Autodesk Inventor part; units mm, degrees
(part 3 of 4)
  spline S198 degree 3 poles (-4.8758, 47.2578) (-4.8804, 47.27) (-4.8822, 47.8237) (-4.8797, 48.4882) knots 0 0 0 0 1 1 1 1
  line L1039 (-4.8758, 47.2578) -> (-4.8804, 47.27) construction
  line L1040 (-4.8804, 47.27) -> (-4.8822, 47.8237) construction
  line L1041 (-4.8822, 47.8237) -> (-4.8797, 48.4882) construction
  line L1042 (-4.8797, 48.4882) -> (-4.8751, 49.6965)
  line L1043 (-4.8751, 49.6965) -> (-4.8001, 49.7019)
  line L1044 (-4.8001, 49.7019) -> (-4.7252, 49.7073)
  line L1045 (-4.7252, 49.7073) -> (-4.7252, 48.5423)
  line L1046 (-4.7252, 48.5423) -> (-4.7252, 47.3772)
  line L1047 (-4.7252, 47.3772) -> (-3.5301, 47.3727)
  line L1048 (-3.5301, 47.3727) -> (-2.3351, 47.3681)
  line L1049 (-2.3351, 47.3681) -> (-2.3351, 47.3064)
  line L1050 (-2.3351, 47.3064) -> (-2.3351, 47.2447)
  line L1051 (-2.3351, 47.2447) -> (-3.6012, 47.2402)
  spline S199 degree 3 poles (-3.6012, 47.2402) (-4.6047, 47.2365) (-4.8691, 47.2402) (-4.8758, 47.2578) knots 11 11 11 11 12 12 12 12
  line L1052 (-3.6012, 47.2402) -> (-4.6047, 47.2365) construction
  line L1053 (-4.6047, 47.2365) -> (-4.8691, 47.2402) construction
  line L1054 (-4.8691, 47.2402) -> (-4.8758, 47.2578) construction
  spline S200 degree 3 poles (-2.2078, 47.2468) (-2.2287, 47.2677) (-2.2232, 49.7053) (-2.2023, 49.7053) (-2.1923, 49.7053) (-2.134, 49.6636) (-2.0728, 49.6127) knots 0 0 0 0 1 1 1 2 2 2 2
  line L1055 (-2.2078, 47.2468) -> (-2.2287, 47.2677) construction
  line L1056 (-2.2287, 47.2677) -> (-2.2232, 49.7053) construction
  line L1057 (-2.2232, 49.7053) -> (-2.2023, 49.7053) construction
  line L1058 (-2.2023, 49.7053) -> (-2.1923, 49.7053) construction
  line L1059 (-2.1923, 49.7053) -> (-2.134, 49.6636) construction
  line L1060 (-2.134, 49.6636) -> (-2.0728, 49.6127) construction
  spline S201 degree 3 poles (-2.0728, 49.6127) (-2.0116, 49.5618) (-1.7837, 49.3794) (-1.5662, 49.2075) knots 2 2 2 2 3 3 3 3
  line L1061 (-2.0728, 49.6127) -> (-2.0116, 49.5618) construction
  line L1062 (-2.0116, 49.5618) -> (-1.7837, 49.3794) construction
  line L1063 (-1.7837, 49.3794) -> (-1.5662, 49.2075) construction
  spline S202 degree 3 poles (-1.5662, 49.2075) (-1.3488, 49.0356) (-1.1154, 48.851) (-1.0475, 48.7972) knots 3 3 3 3 4 4 4 4
  line L1064 (-1.5662, 49.2075) -> (-1.3488, 49.0356) construction
  line L1065 (-1.3488, 49.0356) -> (-1.1154, 48.851) construction
  line L1066 (-1.1154, 48.851) -> (-1.0475, 48.7972) construction
  spline S203 degree 3 poles (-1.0475, 48.7972) (-0.9795, 48.7435) (-0.9144, 48.7016) (-0.9026, 48.7041) knots 4 4 4 4 5 5 5 5
  line L1067 (-1.0475, 48.7972) -> (-0.9795, 48.7435) construction
  line L1068 (-0.9795, 48.7435) -> (-0.9144, 48.7016) construction
  line L1069 (-0.9144, 48.7016) -> (-0.9026, 48.7041) construction
  spline S204 degree 3 poles (-0.9026, 48.7041) (-0.8827, 48.7084) (-0.2139, 49.2329) (0.0269, 49.4331) knots 5 5 5 5 6 6 6 6
  line L1070 (-0.9026, 48.7041) -> (-0.8827, 48.7084) construction
  line L1071 (-0.8827, 48.7084) -> (-0.2139, 49.2329) construction
  line L1072 (-0.2139, 49.2329) -> (0.0269, 49.4331) construction
  spline S205 degree 3 poles (0.0269, 49.4331) (0.2602, 49.6271) (0.373, 49.7068) (0.3818, 49.6839) knots 6 6 6 6 7 7 7 7
  line L1073 (0.0269, 49.4331) -> (0.2602, 49.6271) construction
  line L1074 (0.2602, 49.6271) -> (0.373, 49.7068) construction
  line L1075 (0.373, 49.7068) -> (0.3818, 49.6839) construction
  spline S206 degree 3 poles (0.3818, 49.6839) (0.3865, 49.6714) (0.3884, 49.1175) (0.3859, 48.4529) knots 7 7 7 7 8 8 8 8
  line L1076 (0.3818, 49.6839) -> (0.3865, 49.6714) construction
  line L1077 (0.3865, 49.6714) -> (0.3884, 49.1175) construction
  line L1078 (0.3884, 49.1175) -> (0.3859, 48.4529) construction
  line L1079 (0.3859, 48.4529) -> (0.3813, 47.2447)
  line L1080 (0.3813, 47.2447) -> (0.3196, 47.2447)
  line L1081 (0.3196, 47.2447) -> (0.2578, 47.2447)
  line L1082 (0.2578, 47.2447) -> (0.249, 48.3248)
  line L1083 (0.249, 48.3248) -> (0.2402, 49.4049)
  line L1084 (0.2402, 49.4049) -> (0.0991, 49.2937)
  spline S207 degree 3 poles (0.0991, 49.2937) (-0.7488, 48.6253) (-0.8829, 48.5235) (-0.9156, 48.5235) (-0.9275, 48.5235) (-1.0142, 48.585) (-1.1083, 48.6602) knots 14 14 14 14 15 15 15 16 16 16 16
  line L1085 (0.0991, 49.2937) -> (-0.7488, 48.6253) construction
  line L1086 (-0.7488, 48.6253) -> (-0.8829, 48.5235) construction
  line L1087 (-0.8829, 48.5235) -> (-0.9156, 48.5235) construction
  line L1088 (-0.9156, 48.5235) -> (-0.9275, 48.5235) construction
  line L1089 (-0.9275, 48.5235) -> (-1.0142, 48.585) construction
  line L1090 (-1.0142, 48.585) -> (-1.1083, 48.6602) construction
  spline S208 degree 3 poles (-1.1083, 48.6602) (-1.2024, 48.7354) (-1.3813, 48.8763) (-1.5057, 48.9733) knots 16 16 16 16 17 17 17 17
  line L1091 (-1.1083, 48.6602) -> (-1.2024, 48.7354) construction
  line L1092 (-1.2024, 48.7354) -> (-1.3813, 48.8763) construction
  line L1093 (-1.3813, 48.8763) -> (-1.5057, 48.9733) construction
  spline S209 degree 3 poles (-1.5057, 48.9733) (-1.6302, 49.0703) (-1.8082, 49.2104) (-1.9013, 49.2847) knots 17 17 17 17 18 18 18 18
  line L1094 (-1.5057, 48.9733) -> (-1.6302, 49.0703) construction
  line L1095 (-1.6302, 49.0703) -> (-1.8082, 49.2104) construction
  line L1096 (-1.8082, 49.2104) -> (-1.9013, 49.2847) construction
  line L1097 (-1.9013, 49.2847) -> (-2.0705, 49.4197)
  line L1098 (-2.0705, 49.4197) -> (-2.0793, 48.3322)
  line L1099 (-2.0793, 48.3322) -> (-2.0882, 47.2447)
  line L1100 (-2.0882, 47.2447) -> (-2.1417, 47.2394)
  spline S210 degree 3 poles (-2.1417, 47.2394) (-2.1712, 47.2365) (-2.2009, 47.2398) (-2.2078, 47.2468) knots 22 22 22 22 23 23 23 23
  line L1101 (-2.1417, 47.2394) -> (-2.1712, 47.2365) construction
  line L1102 (-2.1712, 47.2365) -> (-2.2009, 47.2398) construction
  line L1103 (-2.2009, 47.2398) -> (-2.2078, 47.2468) construction
  spline S211 degree 3 poles (0.504, 47.2579) (0.4994, 47.27) (0.4977, 47.8237) (0.5002, 48.4882) knots 0 0 0 0 1 1 1 1
  line L1104 (0.504, 47.2579) -> (0.4994, 47.27) construction
  line L1105 (0.4994, 47.27) -> (0.4977, 47.8237) construction
  line L1106 (0.4977, 47.8237) -> (0.5002, 48.4882) construction
  line L1107 (0.5002, 48.4882) -> (0.5048, 49.6965)
  line L1108 (0.5048, 49.6965) -> (1.7615, 49.701)
  line L1109 (1.7615, 49.701) -> (3.0183, 49.7055)
  line L1110 (3.0183, 49.7055) -> (3.0183, 49.6437)
  spline S212 degree 3 poles (3.0183, 49.6437) (3.0183, 49.6061) (3.0096, 49.5817) (2.9962, 49.5816) knots 5 5 5 5 6 6 6 6
  line L1111 (3.0183, 49.6437) -> (3.0183, 49.6061) construction
  line L1112 (3.0183, 49.6061) -> (3.0096, 49.5817) construction
  line L1113 (3.0096, 49.5817) -> (2.9962, 49.5816) construction
  spline S213 degree 3 poles (2.9962, 49.5816) (2.9841, 49.5814) (2.4444, 49.5816) (1.7968, 49.5818) knots 6 6 6 6 7 7 7 7
  line L1114 (2.9962, 49.5816) -> (2.9841, 49.5814) construction
  line L1115 (2.9841, 49.5814) -> (2.4444, 49.5816) construction
  line L1116 (2.4444, 49.5816) -> (1.7968, 49.5818) construction
  line L1117 (1.7968, 49.5818) -> (0.6194, 49.5823)
  line L1118 (0.6194, 49.5823) -> (0.6194, 49.0617)
  line L1119 (0.6194, 49.0617) -> (0.6194, 48.5411)
  line L1120 (0.6194, 48.5411) -> (1.8188, 48.5411)
  line L1121 (1.8188, 48.5411) -> (3.0183, 48.5411)
  line L1122 (3.0183, 48.5411) -> (3.0183, 48.4813)
  spline S214 degree 3 poles (3.0183, 48.4813) (3.0183, 48.443) (3.0083, 48.4176) (2.9904, 48.4107) knots 13 13 13 13 14 14 14 14
  line L1123 (3.0183, 48.4813) -> (3.0183, 48.443) construction
  line L1124 (3.0183, 48.443) -> (3.0083, 48.4176) construction
  line L1125 (3.0083, 48.4176) -> (2.9904, 48.4107) construction
  spline S215 degree 3 poles (2.9904, 48.4107) (2.9751, 48.4048) (2.4353, 48.4) (1.791, 48.4) knots 14 14 14 14 15 15 15 15
  line L1126 (2.9904, 48.4107) -> (2.9751, 48.4048) construction
  line L1127 (2.9751, 48.4048) -> (2.4353, 48.4) construction
  line L1128 (2.4353, 48.4) -> (1.791, 48.4) construction
  line L1129 (1.791, 48.4) -> (0.6194, 48.4)
  line L1130 (0.6194, 48.4) -> (0.6194, 47.8885)
  line L1131 (0.6194, 47.8885) -> (0.6194, 47.377)
  line L1132 (0.6194, 47.377) -> (1.791, 47.377)
  spline S216 degree 3 poles (1.791, 47.377) (2.4353, 47.377) (2.9751, 47.3721) (2.9904, 47.3663) knots 19 19 19 19 20 20 20 20
  line L1133 (1.791, 47.377) -> (2.4353, 47.377) construction
  line L1134 (2.4353, 47.377) -> (2.9751, 47.3721) construction
  line L1135 (2.9751, 47.3721) -> (2.9904, 47.3663) construction
  spline S217 degree 3 poles (2.9904, 47.3663) (3.0066, 47.36) (3.0183, 47.3349) (3.0183, 47.3064) (3.0183, 47.2779) (3.0066, 47.2528) (2.9904, 47.2466) knots 20 20 20 20 21 21 21 22 22 22 22
  line L1136 (2.9904, 47.3663) -> (3.0066, 47.36) construction
  line L1137 (3.0066, 47.36) -> (3.0183, 47.3349) construction
  line L1138 (3.0183, 47.3349) -> (3.0183, 47.3064) construction
  line L1139 (3.0183, 47.3064) -> (3.0183, 47.2779) construction
  line L1140 (3.0183, 47.2779) -> (3.0066, 47.2528) construction
  line L1141 (3.0066, 47.2528) -> (2.9904, 47.2466) construction
  spline S218 degree 3 poles (2.9904, 47.2466) (2.9751, 47.2407) (2.4112, 47.2359) (1.7375, 47.2359) (0.7737, 47.2359) (0.5107, 47.2405) (0.504, 47.2579) knots 22 22 22 22 23 23 23 24 24 24 24
  line L1142 (2.9904, 47.2466) -> (2.9751, 47.2407) construction
  line L1143 (2.9751, 47.2407) -> (2.4112, 47.2359) construction
  line L1144 (2.4112, 47.2359) -> (1.7375, 47.2359) construction
  line L1145 (1.7375, 47.2359) -> (0.7737, 47.2359) construction
  line L1146 (0.7737, 47.2359) -> (0.5107, 47.2405) construction
  line L1147 (0.5107, 47.2405) -> (0.504, 47.2579) construction
  line L1148 (0.504, 47.2579) -> (0.504, 47.2579)
  spline S219 degree 3 poles (5.3893, 47.496) (5.2553, 47.6391) (5.0332, 47.8753) (4.8957, 48.0208) knots 0 0 0 0 1 1 1 1
  line L1149 (5.3893, 47.496) -> (5.2553, 47.6391) construction
  line L1150 (5.2553, 47.6391) -> (5.0332, 47.8753) construction
  line L1151 (5.0332, 47.8753) -> (4.8957, 48.0208) construction
  spline S220 degree 3 poles (4.8957, 48.0208) (4.7582, 48.1663) (4.6241, 48.3111) (4.5979, 48.3425) knots 1 1 1 1 2 2 2 2
  line L1152 (4.8957, 48.0208) -> (4.7582, 48.1663) construction
  line L1153 (4.7582, 48.1663) -> (4.6241, 48.3111) construction
  line L1154 (4.6241, 48.3111) -> (4.5979, 48.3425) construction
  line L1155 (4.5979, 48.3425) -> (4.5501, 48.3996)
  line L1156 (4.5501, 48.3996) -> (3.8592, 48.4042)
  line L1157 (3.8592, 48.4042) -> (3.1682, 48.4088)
  line L1158 (3.1682, 48.4088) -> (3.1627, 48.475)
  line L1159 (3.1627, 48.475) -> (3.1573, 48.5411)
  line L1160 (3.1573, 48.5411) -> (4.4195, 48.5411)
  line L1161 (4.4195, 48.5411) -> (5.6818, 48.5411)
  line L1162 (5.6818, 48.5411) -> (5.6818, 49.0619)
  line L1163 (5.6818, 49.0619) -> (5.6818, 49.5827)
  line L1164 (5.6818, 49.5827) -> (4.425, 49.5811)
  line L1165 (4.425, 49.5811) -> (3.1682, 49.5796)
  line L1166 (3.1682, 49.5796) -> (3.1627, 49.6424)
  line L1167 (3.1627, 49.6424) -> (3.1573, 49.7053)
  line L1168 (3.1573, 49.7053) -> (4.4813, 49.7053)
  line L1169 (4.4813, 49.7053) -> (5.8052, 49.7053)
  line L1170 (5.8052, 49.7053) -> (5.8052, 49.0634)
  spline S221 degree 3 poles (5.8052, 49.0634) (5.8052, 48.4943) (5.8021, 48.4202) (5.7774, 48.4107) knots 18 18 18 18 19 19 19 19
  line L1171 (5.8052, 49.0634) -> (5.8052, 48.4943) construction
  line L1172 (5.8052, 48.4943) -> (5.8021, 48.4202) construction
  line L1173 (5.8021, 48.4202) -> (5.7774, 48.4107) construction
  spline S222 degree 3 poles (5.7774, 48.4107) (5.762, 48.4048) (5.5191, 48.4) (5.2376, 48.4) knots 19 19 19 19 20 20 20 20
  line L1174 (5.7774, 48.4107) -> (5.762, 48.4048) construction
  line L1175 (5.762, 48.4048) -> (5.5191, 48.4) construction
  line L1176 (5.5191, 48.4) -> (5.2376, 48.4) construction
  line L1177 (5.2376, 48.4) -> (4.7258, 48.4)
  line L1178 (4.7258, 48.4) -> (4.9612, 48.1488)
  spline S223 degree 3 poles (4.9612, 48.1488) (5.0907, 48.0107) (5.3149, 47.7706) (5.4593, 47.6153) knots 22 22 22 22 23 23 23 23
  line L1179 (4.9612, 48.1488) -> (5.0907, 48.0107) construction
  line L1180 (5.0907, 48.0107) -> (5.3149, 47.7706) construction
  line L1181 (5.3149, 47.7706) -> (5.4593, 47.6153) construction
  spline S224 degree 3 poles (5.4593, 47.6153) (5.6037, 47.4599) (5.7402, 47.3157) (5.7627, 47.2947) knots 23 23 23 23 24 24 24 24
  line L1182 (5.4593, 47.6153) -> (5.6037, 47.4599) construction
  line L1183 (5.6037, 47.4599) -> (5.7402, 47.3157) construction
  line L1184 (5.7402, 47.3157) -> (5.7627, 47.2947) construction
  spline S225 degree 3 poles (5.7627, 47.2947) (5.8098, 47.2508) (5.7917, 47.2358) (5.6912, 47.2358) (5.6388, 47.2358) (5.6079, 47.2625) (5.3893, 47.496) knots 24 24 24 24 25 25 25 26 26 26 26
  line L1185 (5.7627, 47.2947) -> (5.8098, 47.2508) construction
  line L1186 (5.8098, 47.2508) -> (5.7917, 47.2358) construction
  line L1187 (5.7917, 47.2358) -> (5.6912, 47.2358) construction
  line L1188 (5.6912, 47.2358) -> (5.6388, 47.2358) construction
  line L1189 (5.6388, 47.2358) -> (5.6079, 47.2625) construction
  line L1190 (5.6079, 47.2625) -> (5.3893, 47.496) construction
  spline S226 degree 3 poles (5.9356, 47.2609) (5.9303, 47.2748) (5.9285, 47.3046) (5.9317, 47.3272) knots 0 0 0 0 1 1 1 1
  line L1191 (5.9356, 47.2609) -> (5.9303, 47.2748) construction
  line L1192 (5.9303, 47.2748) -> (5.9285, 47.3046) construction
  line L1193 (5.9285, 47.3046) -> (5.9317, 47.3272) construction
  line L1194 (5.9317, 47.3272) -> (5.9375, 47.3681)
  line L1195 (5.9375, 47.3681) -> (7.1149, 47.3727)
  line L1196 (7.1149, 47.3727) -> (8.2923, 47.3772)
  line L1197 (8.2923, 47.3772) -> (8.2923, 47.8885)
  line L1198 (8.2923, 47.8885) -> (8.2923, 48.3998)
  line L1199 (8.2923, 48.3998) -> (7.1149, 48.4043)
  line L1200 (7.1149, 48.4043) -> (5.9375, 48.4088)
  line L1201 (5.9375, 48.4088) -> (5.9375, 49.0526)
  line L1202 (5.9375, 49.0526) -> (5.9375, 49.6965)
  line L1203 (5.9375, 49.6965) -> (7.1811, 49.6965)
  line L1204 (7.1811, 49.6965) -> (8.4246, 49.6965)
  line L1205 (8.4246, 49.6965) -> (8.4305, 49.6547)
  spline S227 degree 3 poles (8.4305, 49.6547) (8.4338, 49.6318) (8.4294, 49.606) (8.4207, 49.5973) knots 13 13 13 13 14 14 14 14
  line L1206 (8.4305, 49.6547) -> (8.4338, 49.6318) construction
  line L1207 (8.4338, 49.6318) -> (8.4294, 49.606) construction
  line L1208 (8.4294, 49.606) -> (8.4207, 49.5973) construction
  spline S228 degree 3 poles (8.4207, 49.5973) (8.4118, 49.5884) (7.8969, 49.5816) (7.2374, 49.5816) knots 14 14 14 14 15 15 15 15
  line L1209 (8.4207, 49.5973) -> (8.4118, 49.5884) construction
  line L1210 (8.4118, 49.5884) -> (7.8969, 49.5816) construction
  line L1211 (7.8969, 49.5816) -> (7.2374, 49.5816) construction
  line L1212 (7.2374, 49.5816) -> (6.0698, 49.5815)
  line L1213 (6.0698, 49.5815) -> (6.0698, 49.0615)
  line L1214 (6.0698, 49.0615) -> (6.0698, 48.5414)
  line L1215 (6.0698, 48.5414) -> (7.2472, 48.5368)
  line L1216 (7.2472, 48.5368) -> (8.4246, 48.5323)
  line L1217 (8.4246, 48.5323) -> (8.4246, 47.8885)
  line L1218 (8.4246, 47.8885) -> (8.4246, 47.2447)
  line L1219 (8.4246, 47.2447) -> (7.185, 47.2402)
  spline S229 degree 3 poles (7.185, 47.2402) (6.1218, 47.2363) (5.944, 47.2392) (5.9356, 47.2609) knots 23 23 23 23 24 24 24 24
  line L1220 (7.185, 47.2402) -> (6.1218, 47.2363) construction
  line L1221 (6.1218, 47.2363) -> (5.944, 47.2392) construction
  line L1222 (5.944, 47.2392) -> (5.9356, 47.2609) construction
  spline S230 degree 3 poles (-7.3426, 48.3876) (-7.3645, 48.4036) (-7.3721, 48.4285) (-7.368, 48.4714) knots 0 0 0 0 1 1 1 1
  line L1223 (-7.3426, 48.3876) -> (-7.3645, 48.4036) construction
  line L1224 (-7.3645, 48.4036) -> (-7.3721, 48.4285) construction
  line L1225 (-7.3721, 48.4285) -> (-7.368, 48.4714) construction
  line L1226 (-7.368, 48.4714) -> (-7.3622, 48.5323)
  line L1227 (-7.3622, 48.5323) -> (-6.3127, 48.5323)
  line L1228 (-6.3127, 48.5323) -> (-5.2632, 48.5323)
  line L1229 (-5.2632, 48.5323) -> (-5.2574, 48.4714)
  spline S231 degree 3 poles (-5.2574, 48.4714) (-5.2533, 48.4285) (-5.2609, 48.4036) (-5.2828, 48.3876) knots 5 5 5 5 6 6 6 6
  line L1230 (-5.2574, 48.4714) -> (-5.2533, 48.4285) construction
  line L1231 (-5.2533, 48.4285) -> (-5.2609, 48.4036) construction
  line L1232 (-5.2609, 48.4036) -> (-5.2828, 48.3876) construction
  spline S232 degree 3 poles (-5.2828, 48.3876) (-5.3285, 48.3541) (-7.2968, 48.3541) (-7.3426, 48.3876) knots 6 6 6 6 7 7 7 7
  line L1233 (-5.2828, 48.3876) -> (-5.3285, 48.3541) construction
  line L1234 (-5.3285, 48.3541) -> (-7.2968, 48.3541) construction
  line L1235 (-7.2968, 48.3541) -> (-7.3426, 48.3876) construction
  line L1236 (5.8934, 43.4876) -> (5.8934, 47.0947)
  line L1237 (5.8934, 47.0947) -> (7.1379, 47.0947)
  line L1238 (7.1379, 47.0947) -> (8.3823, 47.0947)
  line L1239 (8.3823, 47.0947) -> (8.7303, 46.7375)
  spline S233 degree 3 poles (8.7303, 46.7375) (8.9217, 46.5411) (9.312, 46.1383) (9.5976, 45.8424) knots 4 4 4 4 5 5 5 5
  line L1240 (8.7303, 46.7375) -> (8.9217, 46.5411) construction
  line L1241 (8.9217, 46.5411) -> (9.312, 46.1383) construction
  line L1242 (9.312, 46.1383) -> (9.5976, 45.8424) construction
  spline S234 degree 3 poles (9.5976, 45.8424) (9.8832, 45.5465) (10.3436, 45.0702) (10.6206, 44.784) knots 5 5 5 5 6 6 6 6
  line L1243 (9.5976, 45.8424) -> (9.8832, 45.5465) construction
  line L1244 (9.8832, 45.5465) -> (10.3436, 45.0702) construction
  line L1245 (10.3436, 45.0702) -> (10.6206, 44.784) construction
  spline S235 degree 3 poles (10.6206, 44.784) (10.8976, 44.4979) (11.227, 44.1565) (11.3525, 44.0256) knots 6 6 6 6 7 7 7 7
  line L1246 (10.6206, 44.784) -> (10.8976, 44.4979) construction
  line L1247 (10.8976, 44.4979) -> (11.227, 44.1565) construction
  line L1248 (11.227, 44.1565) -> (11.3525, 44.0256) construction
  spline S236 degree 3 poles (11.3525, 44.0256) (11.4781, 43.8946) (11.6928, 43.6724) (11.8296, 43.5317) knots 7 7 7 7 8 8 8 8
  line L1249 (11.3525, 44.0256) -> (11.4781, 43.8946) construction
  line L1250 (11.4781, 43.8946) -> (11.6928, 43.6724) construction
  line L1251 (11.6928, 43.6724) -> (11.8296, 43.5317) construction
  spline S237 degree 3 poles (11.8296, 43.5317) (12.7889, 42.5457) (15.1635, 40.0637) (15.2681, 39.9378) knots 8 8 8 8 9 9 9 9
  line L1252 (11.8296, 43.5317) -> (12.7889, 42.5457) construction
  line L1253 (12.7889, 42.5457) -> (15.1635, 40.0637) construction
  line L1254 (15.1635, 40.0637) -> (15.2681, 39.9378) construction
  line L1255 (15.2681, 39.9378) -> (15.3157, 39.8804)
  line L1256 (15.3157, 39.8804) -> (15.0613, 39.8804)
  line L1257 (15.0613, 39.8804) -> (14.8069, 39.8804)
  line L1258 (14.8069, 39.8804) -> (14.4218, 40.2729)
  spline S238 degree 3 poles (14.4218, 40.2729) (14.21, 40.4887) (13.8768, 40.8281) (13.6814, 41.027) knots 13 13 13 13 14 14 14 14
  line L1259 (14.4218, 40.2729) -> (14.21, 40.4887) construction
  line L1260 (14.21, 40.4887) -> (13.8768, 40.8281) construction
  line L1261 (13.8768, 40.8281) -> (13.6814, 41.027) construction
  spline S239 degree 3 poles (13.6814, 41.027) (13.3119, 41.403) (12.256, 42.4917) (10.8884, 43.9067) knots 14 14 14 14 15 15 15 15
  line L1262 (13.6814, 41.027) -> (13.3119, 41.403) construction
  line L1263 (13.3119, 41.403) -> (12.256, 42.4917) construction
  line L1264 (12.256, 42.4917) -> (10.8884, 43.9067) construction
  spline S240 degree 3 poles (10.8884, 43.9067) (10.4499, 44.3603) (10.0773, 44.7457) (10.0605, 44.7631) knots 15 15 15 15 16 16 16 16
  line L1265 (10.8884, 43.9067) -> (10.4499, 44.3603) construction
  line L1266 (10.4499, 44.3603) -> (10.0773, 44.7457) construction
  line L1267 (10.0773, 44.7457) -> (10.0605, 44.7631) construction
  spline S241 degree 3 poles (10.0605, 44.7631) (10.0436, 44.7805) (9.8393, 44.9926) (9.6064, 45.2344) knots 16 16 16 16 17 17 17 17
  line L1268 (10.0605, 44.7631) -> (10.0436, 44.7805) construction
  line L1269 (10.0436, 44.7805) -> (9.8393, 44.9926) construction
  line L1270 (9.8393, 44.9926) -> (9.6064, 45.2344) construction
  spline S242 degree 3 poles (9.6064, 45.2344) (9.1971, 45.6595) (8.828, 46.0412) (8.4256, 46.4552) knots 17 17 17 17 18 18 18 18
  line L1271 (9.6064, 45.2344) -> (9.1971, 45.6595) construction
  line L1272 (9.1971, 45.6595) -> (8.828, 46.0412) construction
  line L1273 (8.828, 46.0412) -> (8.4256, 46.4552) construction
  line L1274 (8.4256, 46.4552) -> (8.2325, 46.6538)
  line L1275 (8.2325, 46.6538) -> (7.2923, 46.6538)
  line L1276 (7.2923, 46.6538) -> (6.352, 46.6538)
  line L1277 (6.352, 46.6538) -> (6.352, 39.8804)
  line L1278 (6.352, 39.8804) -> (6.1227, 39.8804)
  line L1279 (6.1227, 39.8804) -> (5.8934, 39.8804)
  line L1280 (5.8934, 39.8804) -> (5.8934, 43.4876)
  spline S243 degree 3 poles (-5.7835, 40.1295) (-5.9145, 40.2466) (-6.0534, 40.3716) (-6.0922, 40.4073) knots 0 0 0 0 1 1 1 1
  line L1281 (-5.7835, 40.1295) -> (-5.9145, 40.2466) construction
  line L1282 (-5.9145, 40.2466) -> (-6.0534, 40.3716) construction
  line L1283 (-6.0534, 40.3716) -> (-6.0922, 40.4073) construction
  spline S244 degree 3 poles (-6.0922, 40.4073) (-6.131, 40.4429) (-6.4247, 40.7058) (-6.7448, 40.9915) knots 1 1 1 1 2 2 2 2
  line L1284 (-6.0922, 40.4073) -> (-6.131, 40.4429) construction
  line L1285 (-6.131, 40.4429) -> (-6.4247, 40.7058) construction
  line L1286 (-6.4247, 40.7058) -> (-6.7448, 40.9915) construction
  spline S245 degree 3 poles (-6.7448, 40.9915) (-7.065, 41.2771) (-7.3309, 41.5152) (-7.3357, 41.5206) knots 2 2 2 2 3 3 3 3
  line L1287 (-6.7448, 40.9915) -> (-7.065, 41.2771) construction
  line L1288 (-7.065, 41.2771) -> (-7.3309, 41.5152) construction
  line L1289 (-7.3309, 41.5152) -> (-7.3357, 41.5206) construction
  spline S246 degree 3 poles (-7.3357, 41.5206) (-7.3406, 41.526) (-7.4954, 41.665) (-7.6797, 41.8296) knots 3 3 3 3 4 4 4 4
  line L1290 (-7.3357, 41.5206) -> (-7.3406, 41.526) construction
  line L1291 (-7.3406, 41.526) -> (-7.4954, 41.665) construction
  line L1292 (-7.4954, 41.665) -> (-7.6797, 41.8296) construction
  spline S247 degree 3 poles (-7.6797, 41.8296) (-7.864, 41.9942) (-8.1379, 42.2401) (-8.2883, 42.3761) knots 4 4 4 4 5 5 5 5
  line L1293 (-7.6797, 41.8296) -> (-7.864, 41.9942) construction
  line L1294 (-7.864, 41.9942) -> (-8.1379, 42.2401) construction
  line L1295 (-8.1379, 42.2401) -> (-8.2883, 42.3761) construction
  spline S248 degree 3 poles (-8.2883, 42.3761) (-9.4965, 43.468) (-10.4532, 44.3335) (-10.9605, 44.7935) knots 5 5 5 5 6 6 6 6
  line L1296 (-8.2883, 42.3761) -> (-9.4965, 43.468) construction
  line L1297 (-9.4965, 43.468) -> (-10.4532, 44.3335) construction
  line L1298 (-10.4532, 44.3335) -> (-10.9605, 44.7935) construction
  spline S249 degree 3 poles (-10.9605, 44.7935) (-11.2904, 45.0926) (-11.9287, 45.6712) (-12.3791, 46.0793) (-12.8295, 46.4874) (-13.5089, 47.1031) (-13.8889, 47.4475) knots 6 6 6 6 7 7 7 8 8 8 8
  line L1299 (-10.9605, 44.7935) -> (-11.2904, 45.0926) construction
  line L1300 (-11.2904, 45.0926) -> (-11.9287, 45.6712) construction
  line L1301 (-11.9287, 45.6712) -> (-12.3791, 46.0793) construction
  line L1302 (-12.3791, 46.0793) -> (-12.8295, 46.4874) construction
  line L1303 (-12.8295, 46.4874) -> (-13.5089, 47.1031) construction
  line L1304 (-13.5089, 47.1031) -> (-13.8889, 47.4475) construction
  spline S250 degree 3 poles (-13.8889, 47.4475) (-14.2688, 47.7919) (-14.9696, 48.4269) (-15.4461, 48.8586) knots 8 8 8 8 9 9 9 9
  line L1305 (-13.8889, 47.4475) -> (-14.2688, 47.7919) construction
  line L1306 (-14.2688, 47.7919) -> (-14.9696, 48.4269) construction
  line L1307 (-14.9696, 48.4269) -> (-15.4461, 48.8586) construction
  line L1308 (-15.4461, 48.8586) -> (-16.3125, 49.6436)
  line L1309 (-16.3125, 49.6436) -> (-16.0479, 49.6484)
  spline S251 degree 3 poles (-16.0479, 49.6484) (-15.9024, 49.6511) (-15.7726, 49.6472) (-15.7596, 49.6396) knots 11 11 11 11 12 12 12 12
  line L1310 (-16.0479, 49.6484) -> (-15.9024, 49.6511) construction
  line L1311 (-15.9024, 49.6511) -> (-15.7726, 49.6472) construction
  line L1312 (-15.7726, 49.6472) -> (-15.7596, 49.6396) construction
  spline S252 degree 3 poles (-15.7596, 49.6396) (-15.7369, 49.6265) (-15.1884, 49.1406) (-13.9415, 48.0294) knots 12 12 12 12 13 13 13 13
  line L1313 (-15.7596, 49.6396) -> (-15.7369, 49.6265) construction
  line L1314 (-15.7369, 49.6265) -> (-15.1884, 49.1406) construction
  line L1315 (-15.1884, 49.1406) -> (-13.9415, 48.0294) construction
  spline S253 degree 3 poles (-13.9415, 48.0294) (-13.6213, 47.744) (-13.2736, 47.4329) (-13.1688, 47.3379) knots 13 13 13 13 14 14 14 14
  line L1316 (-13.9415, 48.0294) -> (-13.6213, 47.744) construction
  line L1317 (-13.6213, 47.744) -> (-13.2736, 47.4329) construction
  line L1318 (-13.2736, 47.4329) -> (-13.1688, 47.3379) construction
  spline S254 degree 3 poles (-13.1688, 47.3379) (-13.064, 47.243) (-12.9211, 47.1166) (-12.8513, 47.0571) knots 14 14 14 14 15 15 15 15
  line L1319 (-13.1688, 47.3379) -> (-13.064, 47.243) construction
  line L1320 (-13.064, 47.243) -> (-12.9211, 47.1166) construction
  line L1321 (-12.9211, 47.1166) -> (-12.8513, 47.0571) construction
  spline S255 degree 3 poles (-12.8513, 47.0571) (-12.7815, 46.9976) (-12.6887, 46.916) (-12.645, 46.8759) knots 15 15 15 15 16 16 16 16
  line L1322 (-12.8513, 47.0571) -> (-12.7815, 46.9976) construction
  line L1323 (-12.7815, 46.9976) -> (-12.6887, 46.916) construction
  line L1324 (-12.6887, 46.916) -> (-12.645, 46.8759) construction
  spline S256 degree 3 poles (-12.645, 46.8759) (-12.5636, 46.8011) (-12.1786, 46.4566) (-11.9828, 46.2833) knots 16 16 16 16 17 17 17 17
  line L1325 (-12.645, 46.8759) -> (-12.5636, 46.8011) construction
  line L1326 (-12.5636, 46.8011) -> (-12.1786, 46.4566) construction
  line L1327 (-12.1786, 46.4566) -> (-11.9828, 46.2833) construction
  spline S257 degree 3 poles (-11.9828, 46.2833) (-11.8512, 46.1668) (-11.598, 45.9399) (-11.3927, 45.7542) knots 17 17 17 17 18 18 18 18
  line L1328 (-11.9828, 46.2833) -> (-11.8512, 46.1668) construction
  line L1329 (-11.8512, 46.1668) -> (-11.598, 45.9399) construction
  line L1330 (-11.598, 45.9399) -> (-11.3927, 45.7542) construction
  spline S258 degree 3 poles (-11.3927, 45.7542) (-11.3102, 45.6796) (-11.1594, 45.5443) (-11.0575, 45.4535) knots 18 18 18 18 19 19 19 19
  line L1331 (-11.3927, 45.7542) -> (-11.3102, 45.6796) construction
  line L1332 (-11.3102, 45.6796) -> (-11.1594, 45.5443) construction
  line L1333 (-11.1594, 45.5443) -> (-11.0575, 45.4535) construction
  spline S259 degree 3 poles (-11.0575, 45.4535) (-10.9557, 45.3627) (-10.6779, 45.1137) (-10.4402, 44.9003) knots 19 19 19 19 20 20 20 20
  line L1334 (-11.0575, 45.4535) -> (-10.9557, 45.3627) construction
  line L1335 (-10.9557, 45.3627) -> (-10.6779, 45.1137) construction
  line L1336 (-10.6779, 45.1137) -> (-10.4402, 44.9003) construction
  spline S260 degree 3 poles (-10.4402, 44.9003) (-10.2025, 44.6868) (-9.8969, 44.4127) (-9.7611, 44.2911) knots 20 20 20 20 21 21 21 21
  line L1337 (-10.4402, 44.9003) -> (-10.2025, 44.6868) construction
  line L1338 (-10.2025, 44.6868) -> (-9.8969, 44.4127) construction
  line L1339 (-9.8969, 44.4127) -> (-9.7611, 44.2911) construction
  spline S261 degree 3 poles (-9.7611, 44.2911) (-9.6253, 44.1695) (-9.5102, 44.0658) (-9.5053, 44.0605) knots 21 21 21 21 22 22 22 22
  line L1340 (-9.7611, 44.2911) -> (-9.6253, 44.1695) construction
  line L1341 (-9.6253, 44.1695) -> (-9.5102, 44.0658) construction
  line L1342 (-9.5102, 44.0658) -> (-9.5053, 44.0605) construction
  spline S262 degree 3 poles (-9.5053, 44.0605) (-9.5005, 44.0553) (-9.306, 43.8811) (-9.0731, 43.6734) knots 22 22 22 22 23 23 23 23
  line L1343 (-9.5053, 44.0605) -> (-9.5005, 44.0553) construction
  line L1344 (-9.5005, 44.0553) -> (-9.306, 43.8811) construction
  line L1345 (-9.306, 43.8811) -> (-9.0731, 43.6734) construction
  spline S263 degree 3 poles (-9.0731, 43.6734) (-8.8403, 43.4657) (-8.606, 43.2556) (-8.5525, 43.2065) knots 23 23 23 23 24 24 24 24
  line L1346 (-9.0731, 43.6734) -> (-8.8403, 43.4657) construction
  line L1347 (-8.8403, 43.4657) -> (-8.606, 43.2556) construction
  line L1348 (-8.606, 43.2556) -> (-8.5525, 43.2065) construction
  spline S264 degree 3 poles (-8.5525, 43.2065) (-8.499, 43.1574) (-8.3879, 43.057) (-8.3056, 42.9834) knots 24 24 24 24 25 25 25 25
  line L1349 (-8.5525, 43.2065) -> (-8.499, 43.1574) construction
  line L1350 (-8.499, 43.1574) -> (-8.3879, 43.057) construction
  line L1351 (-8.3879, 43.057) -> (-8.3056, 42.9834) construction
  spline S265 degree 3 poles (-8.3056, 42.9834) (-8.1563, 42.8499) (-7.7078, 42.4478) (-7.4243, 42.1931) knots 25 25 25 25 26 26 26 26
  line L1352 (-8.3056, 42.9834) -> (-8.1563, 42.8499) construction
  line L1353 (-8.1563, 42.8499) -> (-7.7078, 42.4478) construction
  line L1354 (-7.7078, 42.4478) -> (-7.4243, 42.1931) construction
  spline S266 degree 3 poles (-7.4243, 42.1931) (-7.3421, 42.1193) (-7.2267, 42.0152) (-7.1679, 41.9618) knots 26 26 26 26 27 27 27 27
  line L1355 (-7.4243, 42.1931) -> (-7.3421, 42.1193) construction
  line L1356 (-7.3421, 42.1193) -> (-7.2267, 42.0152) construction
  line L1357 (-7.2267, 42.0152) -> (-7.1679, 41.9618) construction
  spline S267 degree 3 poles (-7.1679, 41.9618) (-7.1091, 41.9085) (-6.9938, 41.8046) (-6.9117, 41.731) knots 27 27 27 27 28 28 28 28
  line L1358 (-7.1679, 41.9618) -> (-7.1091, 41.9085) construction
  line L1359 (-7.1091, 41.9085) -> (-6.9938, 41.8046) construction
  line L1360 (-6.9938, 41.8046) -> (-6.9117, 41.731) construction
  spline S268 degree 3 poles (-6.9117, 41.731) (-6.8296, 41.6575) (-6.5912, 41.4432) (-6.382, 41.2548) knots 28 28 28 28 29 29 29 29
  line L1361 (-6.9117, 41.731) -> (-6.8296, 41.6575) construction
  line L1362 (-6.8296, 41.6575) -> (-6.5912, 41.4432) construction
  line L1363 (-6.5912, 41.4432) -> (-6.382, 41.2548) construction
  spline S269 degree 3 poles (-6.382, 41.2548) (-5.6688, 40.6128) (-5.5691, 40.5242) (-5.5528, 40.5184) knots 29 29 29 29 30 30 30 30
  line L1364 (-6.382, 41.2548) -> (-5.6688, 40.6128) construction
  line L1365 (-5.6688, 40.6128) -> (-5.5691, 40.5242) construction
  line L1366 (-5.5691, 40.5242) -> (-5.5528, 40.5184) construction
  spline S270 degree 3 poles (-5.5528, 40.5184) (-5.5429, 40.5148) (-5.5366, 41.8055) (-5.5366, 43.8213) (-5.5366, 43.8213) (-5.5366, 47.1267) (-5.5366, 47.13) knots 30 30 30 30 31 31 31 32 32 32 32
  line L1367 (-5.5528, 40.5184) -> (-5.5429, 40.5148) construction
  line L1368 (-5.5429, 40.5148) -> (-5.5366, 41.8055) construction
  line L1369 (-5.5366, 41.8055) -> (-5.5366, 43.8213) construction
  line L1370 (-5.5366, 43.8213) -> (-5.5366, 43.8213) construction
  line L1371 (-5.5366, 43.8213) -> (-5.5366, 47.13) construction
  line L1372 (-5.5366, 47.13) -> (-5.5366, 47.13) construction
  line L1373 (-5.5366, 47.13) -> (-5.2808, 47.13)
  line L1374 (-5.2808, 47.13) -> (-5.025, 47.13)
  line L1375 (-5.025, 47.13) -> (-5.025, 39.9157)
  line L1376 (-5.025, 39.9157) -> (-5.2852, 39.9161)
  line L1377 (-5.2852, 39.9161) -> (-5.5454, 39.9165)
  line L1378 (-5.5454, 39.9165) -> (-5.7835, 40.1295)
  spline S271 degree 3 poles (5.2849, 42.5564) (5.2558, 42.5718) (5.1288, 42.6808) (5.0027, 42.7985) knots 0 0 0 0 1 1 1 1
  line L1379 (5.2849, 42.5564) -> (5.2558, 42.5718) construction
  line L1380 (5.2558, 42.5718) -> (5.1288, 42.6808) construction
  line L1381 (5.1288, 42.6808) -> (5.0027, 42.7985) construction
  spline S272 degree 3 poles (5.0027, 42.7985) (4.757, 43.0278) (4.1431, 43.5913) (3.6268, 44.0614) knots 1 1 1 1 2 2 2 2
  line L1382 (5.0027, 42.7985) -> (4.757, 43.0278) construction
  line L1383 (4.757, 43.0278) -> (4.1431, 43.5913) construction
  line L1384 (4.1431, 43.5913) -> (3.6268, 44.0614) construction
  spline S273 degree 3 poles (3.6268, 44.0614) (3.4522, 44.2204) (3.2465, 44.4084) (3.1697, 44.4791) knots 2 2 2 2 3 3 3 3
  line L1385 (3.6268, 44.0614) -> (3.4522, 44.2204) construction
  line L1386 (3.4522, 44.2204) -> (3.2465, 44.4084) construction
  line L1387 (3.2465, 44.4084) -> (3.1697, 44.4791) construction
  line L1388 (3.1697, 44.4791) -> (3.0301, 44.6076)
  line L1389 (3.0301, 44.6076) -> (1.7718, 44.6076)
  line L1390 (1.7718, 44.6076) -> (0.5136, 44.6076)
  line L1391 (0.5136, 44.6076) -> (0.5136, 44.8281)
  line L1392 (0.5136, 44.8281) -> (0.5136, 45.0486)
  line L1393 (0.5136, 45.0486) -> (2.9125, 45.0486)
  line L1394 (2.9125, 45.0486) -> (5.3113, 45.0486)
  line L1395 (5.3113, 45.0486) -> (5.3113, 45.8688)
  line L1396 (5.3113, 45.8688) -> (5.3113, 46.689)
  line L1397 (5.3113, 46.689) -> (2.9125, 46.689)
  line L1398 (2.9125, 46.689) -> (0.5136, 46.689)
  line L1399 (0.5136, 46.689) -> (0.5136, 46.9007)
  line L1400 (0.5136, 46.9007) -> (0.5136, 47.1124)
  line L1401 (0.5136, 47.1124) -> (5.7523, 47.1124)
  line L1402 (5.7523, 47.1124) -> (5.7523, 45.8602)
  line L1403 (5.7523, 45.8602) -> (5.7523, 44.6079)
  line L1404 (5.7523, 44.6079) -> (4.7417, 44.6034)
  line L1405 (4.7417, 44.6034) -> (3.7311, 44.5988)
  line L1406 (3.7311, 44.5988) -> (4.0494, 44.3033)
  spline S274 degree 3 poles (4.0494, 44.3033) (4.2244, 44.1407) (4.4034, 43.9738) (4.447, 43.9323) knots 23 23 23 23 24 24 24 24
  line L1407 (4.0494, 44.3033) -> (4.2244, 44.1407) construction
  line L1408 (4.2244, 44.1407) -> (4.4034, 43.9738) construction
  line L1409 (4.4034, 43.9738) -> (4.447, 43.9323) construction
  spline S275 degree 3 poles (4.447, 43.9323) (4.4907, 43.8909) (4.5899, 43.7984) (4.6675, 43.7268) knots 24 24 24 24 25 25 25 25
  line L1410 (4.447, 43.9323) -> (4.4907, 43.8909) construction
  line L1411 (4.4907, 43.8909) -> (4.5899, 43.7984) construction
  line L1412 (4.5899, 43.7984) -> (4.6675, 43.7268) construction
  spline S276 degree 3 poles (4.6675, 43.7268) (4.7451, 43.6552) (4.8642, 43.544) (4.9321, 43.4796) knots 25 25 25 25 26 26 26 26
  line L1413 (4.6675, 43.7268) -> (4.7451, 43.6552) construction
  line L1414 (4.7451, 43.6552) -> (4.8642, 43.544) construction
  line L1415 (4.8642, 43.544) -> (4.9321, 43.4796) construction
  spline S277 degree 3 poles (4.9321, 43.4796) (5, 43.4151) (5.2001, 43.2295) (5.3768, 43.0671) knots 26 26 26 26 27 27 27 27
  line L1416 (4.9321, 43.4796) -> (5, 43.4151) construction
  line L1417 (5, 43.4151) -> (5.2001, 43.2295) construction
  line L1418 (5.2001, 43.2295) -> (5.3768, 43.0671) construction
  spline S278 degree 3 poles (5.3768, 43.0671) (5.5534, 42.9047) (5.7142, 42.7491) (5.734, 42.7213) knots 27 27 27 27 28 28 28 28
  line L1419 (5.3768, 43.0671) -> (5.5534, 42.9047) construction
  line L1420 (5.5534, 42.9047) -> (5.7142, 42.7491) construction
  line L1421 (5.7142, 42.7491) -> (5.734, 42.7213) construction
  spline S279 degree 3 poles (5.734, 42.7213) (5.7542, 42.693) (5.77, 42.6429) (5.77, 42.6073) knots 28 28 28 28 29 29 29 29
  line L1422 (5.734, 42.7213) -> (5.7542, 42.693) construction
  line L1423 (5.7542, 42.693) -> (5.77, 42.6429) construction
  line L1424 (5.77, 42.6429) -> (5.77, 42.6073) construction
  line L1425 (5.77, 42.6073) -> (5.77, 42.5439)
  line L1426 (5.77, 42.5439) -> (5.6156, 42.5437)
  spline S280 degree 3 poles (5.6156, 42.5437) (5.5307, 42.5436) (5.4335, 42.5401) (5.3995, 42.5359) knots 31 31 31 31 32 32 32 32
  line L1427 (5.6156, 42.5437) -> (5.5307, 42.5436) construction
  line L1428 (5.5307, 42.5436) -> (5.4335, 42.5401) construction
  line L1429 (5.4335, 42.5401) -> (5.3995, 42.5359) construction
  spline S281 degree 3 poles (5.3995, 42.5359) (5.3632, 42.5314) (5.3161, 42.5399) (5.2849, 42.5564) knots 32 32 32 32 33 33 33 33
  line L1430 (5.3995, 42.5359) -> (5.3632, 42.5314) construction
  line L1431 (5.3632, 42.5314) -> (5.3161, 42.5399) construction
  line L1432 (5.3161, 42.5399) -> (5.2849, 42.5564) construction
  line L1433 (-4.8839, 44.8281) -> (-4.8839, 47.1124)
  line L1434 (-4.8839, 47.1124) -> (-2.2557, 47.1124)
  line L1435 (-2.2557, 47.1124) -> (0.3725, 47.1124)
  line L1436 (0.3725, 47.1124) -> (0.3725, 46.9007)
  line L1437 (0.3725, 46.9007) -> (0.3725, 46.689)
  line L1438 (0.3725, 46.689) -> (-2.0352, 46.689)
  line L1439 (-2.0352, 46.689) -> (-4.443, 46.689)
  line L1440 (-4.443, 46.689) -> (-4.443, 45.8688)
  line L1441 (-4.443, 45.8688) -> (-4.443, 45.0486)
  line L1442 (-4.443, 45.0486) -> (-2.0352, 45.0486)
  line L1443 (-2.0352, 45.0486) -> (0.3725, 45.0486)
  line L1444 (0.3725, 45.0486) -> (0.3725, 44.8281)
  line L1445 (0.3725, 44.8281) -> (0.3725, 44.6076)
  line L1446 (0.3725, 44.6076) -> (-2.0352, 44.6076)
  line L1447 (-2.0352, 44.6076) -> (-4.443, 44.6076)
  line L1448 (-4.443, 44.6076) -> (-4.443, 43.7963)
  line L1449 (-4.443, 43.7963) -> (-4.443, 42.9849)
  line L1450 (-4.443, 42.9849) -> (-2.0352, 42.9849)
  line L1451 (-2.0352, 42.9849) -> (0.3725, 42.9849)
  line L1452 (0.3725, 42.9849) -> (0.3725, 42.7644)
  line L1453 (0.3725, 42.7644) -> (0.3725, 42.5439)
  line L1454 (0.3725, 42.5439) -> (-2.2557, 42.5439)
  line L1455 (-2.2557, 42.5439) -> (-4.8839, 42.5439)
  line L1456 (-4.8839, 42.5439) -> (-4.8839, 44.8281)
  line L1457 (6.5637, 42.7556) -> (6.5637, 42.9672)
  line L1458 (6.5637, 42.9672) -> (9.0541, 42.9672)
  line L1459 (9.0541, 42.9672) -> (11.5445, 42.9672)
  line L1460 (11.5445, 42.9672) -> (11.7124, 42.8041)
  spline S282 degree 3 poles (11.7124, 42.8041) (11.8047, 42.7143) (11.8992, 42.6191) (11.9223, 42.5924) knots 4 4 4 4 5 5 5 5
  line L1461 (11.7124, 42.8041) -> (11.8047, 42.7143) construction
  line L1462 (11.8047, 42.7143) -> (11.8992, 42.6191) construction
  line L1463 (11.8992, 42.6191) -> (11.9223, 42.5924) construction
  line L1464 (11.9223, 42.5924) -> (11.9643, 42.5439)
  line L1465 (11.9643, 42.5439) -> (9.264, 42.5439)
  line L1466 (9.264, 42.5439) -> (6.5637, 42.5439)
  line L1467 (6.5637, 42.5439) -> (6.5637, 42.7556)
  point P0 (0, 0)
  constraints: 542 end point, 817 other
sketch "Sketch3" plane through (0, 0, 5) normal (0, 0, 1) x (1, 0, 0)
  line L0 (0, -39.5) -> (0, 79.5) construction
  circle A0 centre (67.5, -16.5) radius 1.5
  circle A1 centre (47, 36) radius 1.5
  circle A2 centre (-67.5, -16.5) radius 1.5
  circle A3 centre (-47, 36) radius 1.5
  line L1 (-75, -22.5) -> (75, -22.5) projected
  point P0 (0, 0)
  dimension "d5" = 3
  dimension "d6" = 3
  dimension "d7" = 94
  dimension "d8" = 135
  dimension "d9" = 6
  dimension "d10" = 52.5
  constraints: 4 centre point, 2 symmetric about line, 2 other
  measures "d5" diameter of A0
  measures "d6" diameter of A1
  measures "d7" distance of A1.centre A3.centre
  measures "d8" distance of A2.centre A0.centre
  measures "d9" distance from line of L1 A0.centre
  measures "d10" vertical distance of A0.centre A1.centre
extrude "Extrusion2" cut sketch "Sketch3" against normal up to next
sketch "Sketch4" plane through (0, 0, 5) normal (0, 0, 1) x (1, 0, 0)
  circle A0 centre (-47, 36) radius 1.5 projected
  circle A1 centre (-47, 36) radius 3
  circle A2 centre (47, 36) radius 3
  circle A3 centre (67.5, -16.5) radius 1.5 projected
  circle A4 centre (67.5, -16.5) radius 3
  circle A5 centre (-67.5, -16.5) radius 3
  circle A6 centre (-67.5, -16.5) radius 1.5 projected
  circle A7 centre (47, 36) radius 1.5 projected
  point P0 (0, 0)
  dimension "d20" = 6
  dimension "d21" = 6
  dimension "d22" = 6
  dimension "d23" = 6
  constraints: 4 centre point, 2 coincident, 2 concentric
  measures "d20" diameter of A1
  measures "d21" diameter of A2
  measures "d22" diameter of A5
  measures "d23" diameter of A4
extrude "Extrusion3" cut sketch "Sketch4" against normal blind 3 contours A1 | A2 | A4 | A5 | A6
sketch "Sketch5" plane through (0, 0, 5) normal (0, 0, 1) x (1, 0, 0)
  line L0 (-57, -7.5) -> (-22, -7.5)
  line L1 (-22, -7.5) -> (-22, 15)
  line L2 (-22, 15) -> (-57, 15)
  line L3 (-57, 15) -> (-57, -7.5)
  line L4 (-57, -7.5) -> (-22, 15) construction
  line L5 (-22, -7.5) -> (-57, 15) construction
  line L6 (-22, 2.2127) -> (-22, 8.5968)
  line L7 (-57, 2.2127) -> (-57, 8.5968)
  line L8 (-67.1067, 3.75) -> (-18.4073, 3.75) construction
  line L9 (-39.5, -12.5176) -> (-39.5, 24.13) construction
  line L10 (-22, -1.75) -> (-19, -1.75)
  line L11 (-19, -1.75) -> (-19, 9.25)
  line L12 (-19, 9.25) -> (-22, 9.25)
  line L13 (-22, 9.25) -> (-22, -1.75)
  line L14 (-22, -1.75) -> (-19, 9.25) construction
  line L15 (-19, -1.75) -> (-22, 9.25) construction
  line L16 (-57, -1.75) -> (-60, -1.75)
  line L17 (-60, -1.75) -> (-60, 9.25)
  line L18 (-60, 9.25) -> (-57, 9.25)
  line L19 (-57, 9.25) -> (-57, -1.75)
  line L20 (-57, -1.75) -> (-60, 9.25) construction
  line L21 (-60, -1.75) -> (-57, 9.25) construction
  line L22 (-75, -22.5) -> (75, -22.5) projected
  line L23 (-75, 22.5) -> (-75, -22.5) projected
  point P0 (0, 0)
  point P1 (-39.5, 3.75)
  point P2 (-20.5, 3.75)
  point P3 (-58.5, 3.75)
  dimension "d26" = 22.5
  dimension "d27" = 35
  dimension "d29" = 41
  dimension "d30" = 11
  dimension "d31" = 15
  dimension "d32" = 15
  constraints: 44 end point, 6 midpoint, 5 symmetric about line, 4 parallel, 3 horizontal, 3 point on line, 2 perpendicular, 1 collinear, 1 vertical, 2 other
  measures "d26" distance between parallel lines of L0 L2
  measures "d27" distance between parallel lines of L3 L1
  measures "d29" distance between parallel lines of L17 L11
  measures "d30" distance between parallel lines of L12 L10
  measures "d31" distance between parallel lines of L22 L0
  measures "d32" distance between parallel lines of L17 L23
extrude "Extrusion4" cut sketch "Sketch5" against normal up to next
sketch "Sketch6" plane through (0, 0, 5) normal (0, 0, 1) x (1, 0, 0)
  line L0 (-67.1067, 3.75) -> (-18.4073, 3.75) construction
  line L1 (-51.0918, 3.75) -> (-31.6555, 3.75) construction
  line L2 (-39.5, -12.5176) -> (-39.5, 24.13) construction
  point P0 (0, 0)
  point P1 (-14.5, 3.75)
  point P2 (-64.5, 3.75)
  dimension "d35" = 50
  constraints: 3 point on line, 2 end point, 1 symmetric about line
  measures "d35" distance of point (-14.5, 3.75) point (-64.5, 3.75)
hole "Hole2" at (-64.5, 3.75, 5) at (-14.5, 3.75, 5) direction (0, 0, -1) diameter 3 end through all counterbore diameter 6 counterbore depth 3
sketch "Sketch7" plane through (0, 0, 5) normal (0, 0, 1) x (1, 0, 0)
  line L0 (-6.4691, -17.5) -> (23.5309, -17.5)
  line L1 (23.5309, -17.5) -> (23.5309, 17.5)
  line L2 (23.5309, 17.5) -> (-6.4691, 17.5)
  line L3 (-6.4691, 17.5) -> (-6.4691, -17.5)
  line L4 (-6.4691, -17.5) -> (23.5309, 17.5) construction
  line L5 (23.5309, -17.5) -> (-6.4691, 17.5) construction
  line L6 (-105, 0) -> (105, 0) construction
  point P0 (0, 0)
  point P1 (8.5309, 0)
  point P2 (8.5309, 0)
  dimension "d43" = 30
  dimension "d44" = 35
  constraints: 12 end point, 3 midpoint, 2 parallel, 1 horizontal, 1 perpendicular, 1 point on line
  measures "d43" distance of L1.end L2.end
  measures "d44" distance of L0.end L1.end
extrude "Extrusion5" cut sketch "Sketch7" against normal up to next
fillet "Fillet1" radius 0.4 12 edges at (-57, 9.25, 2.5) (-22, 15, 2.5) (-19, 9.25, 2.5) (-22, 9.25, 2.5) (-19, -1.75, 2.5) (-22, -1.75, 2.5) (-22, -7.5, 2.5) (-57, -7.5, 2.5) (-57, -1.75, 2.5) (-60, -1.75, 2.5) (-60, 9.25, 2.5) (-57, 15, 2.5)
fillet "Fillet1" radius 5.25 4 edges at (23.5309, 17.5, 2.5) (23.5309, -17.5, 2.5) (-6.4691, -17.5, 2.5) (-6.4691, 17.5, 2.5)
fillet "Fillet2" radius 10 4 edges at (-75, -22.5, 2.5) (75, 22.5, 2.5) (75, -22.5, 2.5) (-75, 22.5, 2.5)
chamfer "Chamfer1" distance 0.2 angle 45 46 edges at (0, -22.5, 0) (-72.0711, -19.5711, 0) (-75, 3.4292, 0) (-74.5114, 22.446, 0) (0, 62.5, 0) (74.5114, 22.446, 0) (75, 3.4292, 0) (72.0711, -19.5711, 0) (-39.5, -7.5, 0) (-22.1172, -7.3828, 0) (-22, -4.625, 0) (-21.8828, -1.8672, 0) (-20.5, -1.75, 0) (-19.1172, -1.6328, 0) (-19, 3.75, 0) (-19.1172, 9.1328, 0) (-20.5, 9.25, 0) (-21.8828, 9.3672, 0) (-22, 12.125, 0) (-22.1172, 14.8828, 0) (-39.5, 15, 0) (-56.8828, 14.8828, 0) (-57, 12.125, 0) (-57.1172, 9.3672, 0) (-58.5, 9.25, 0) (-59.8828, 9.1328, 0) (-60, 3.75, 0) (-59.8828, -1.6328, 0) (-58.5, -1.75, 0) (-57.1172, -1.8672, 0) (-57, -4.625, 0) (-56.8828, -7.3828, 0) (-69, -16.5, 0) (-64.5, 5.25, 0) (-48.5, 36, 0) (-14.5, 5.25, 0) (-6.4691, 0, 0) (-4.9315, -15.9623, 0) (8.5309, -17.5, 0) (21.9932, -15.9623, 0) (23.5309, 0, 0) (21.9932, 15.9623, 0) (8.5309, 17.5, 0) (-4.9315, 15.9623, 0) (66, -16.5, 0) (45.5, 36, 0)